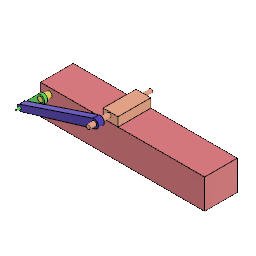
4 v1 (Autodesk Fusion 360 design; units mm, degrees)
Autodesk Fusion 360 part; units mm, degrees
sketch "Sketch1" plane through (0, 0, 0) normal (0, 1, 0) x (1, 0, 0)
  line L0 (0, -50) -> (150, -50)
  line L1 (150, -50) -> (150, 0)
  line L2 (150, 0) -> (0, 0)
  line L3 (0, 0) -> (0, -50)
  line L4 (125, -50) -> (150, -50)
  line L5 (150, -50) -> (150, -65)
  line L6 (150, -65) -> (125, -65)
  line L7 (125, -65) -> (125, -50)
  circle A0 centre (135, -60) radius 3.3426
  circle A1 centre (15, -40) radius 4.5426
  constraint horizontal L0
  constraint vertical L1
  constraint horizontal L2
  constraint vertical L3
  constraint horizontal L4
  constraint vertical L5
  constraint horizontal L6
  constraint vertical L7
  constraint coincident L0 L4.start
extrude "Extrude1" add sketch "Sketch1" along normal blind 55 contours L0 L1 L2 L3 L4 makes body 1 in component "Component"
extrude "Extrude1'" add sketch "Sketch1" along normal blind 55 separate body contours L0 L4 L5 L6 L7 makes body 2 in component "Component'"
extrude "Extrude1''" add sketch "Sketch1" along normal blind 60 and the other way blind 10 separate body contours A1 makes body 3 in component "Component''"
sketch "Sketch2" plane through (0, -10, 0) normal (0, -1, 0) x (1, 0, 0)
  circle A0 centre (15, 40) radius 4.5426
  circle A1 centre (15, 40) radius 7.2111
  circle A2 centre (15, 8.7998) radius 3.3899
  line L0 (7.8047, 40.4772) -> (11.634, 8.398)
  line L1 (22.1953, 40.4772) -> (18.366, 8.398)
  constraint concentric A0 A1
  constraint coincident A1 L0.start
  constraint coincident A2 L0.end
  constraint tangent A2 L0
  constraint coincident A1 L1.start
  constraint coincident A2 L1.end
  constraint tangent A2 L1
sketch "Sketch3" plane through (0, -10, 0) normal (0, -1, 0) x (1, 0, 0)
  circle A0 centre (15, 9) radius 1.6144
extrude "Extrude1'''" add sketch "Sketch2" along normal blind 5 separate body contours A1 L0 L1 | A1 A2 L0 L1 | A2 makes body 4 in component "Component'''"
extrude "Extrude2" cut sketch "Sketch3" along normal blind 10 bodies 4 in component "Component'''"
sketch "Sketch4" plane through (0, 0, 0) normal (0, 1, 0) x (1, 0, 0)
  circle A0 centre (135, -60) radius 80.8968
sketch "Sketch5" plane through (0, 0, 0) normal (0, 1, 0) x (1, 0, 0)
  circle A0 centre (135, -60) radius 7.074
  circle A1 centre (15, -9) radius 2.2361
  circle A2 centre (15, -9) radius 5.099
  circle A3 centre (135, -60) radius 4.1231
  line L0 (12.9347, -13.662) -> (132.1348, -66.4678)
  line L1 (137.668, -53.4484) -> (16.9231, -4.2775)
  constraint concentric A1 A2
  constraint concentric A0 A3
  constraint coincident A2 L0.start
  constraint coincident A0 L0.end
  constraint coincident A0 L1.start
  constraint coincident A2 L1.end
  constraint tangent A2 L1
  constraint tangent A0 L1
  constraint tangent A0 L0
  constraint tangent A2 L0
extrude "Extrude1''''" add sketch "Sketch5" along normal blind 10 separate body makes body 5
move_body "Move1" bodies 5 to x (1, 0, 0) y (0, 1, 0) z (0, 0, 1) at (0, -25, 0)
copy_body "Body->Comp1" bodies 5 removing the originals makes body 6 in component "Component''''"
extrude "Extrude2'" add sketch "Sketch1" along normal blind 70 and the other way blind 35 contours A0 bodies 2 in component "Component'"
extrude "Extrude3" add sketch "Sketch3" along normal blind 15 bodies 4 in component "Component'''"
extrude "Extrude4" add 1 faces at (15.4446, -25, 8.6969) along direction (0, -1, 0) blind 6.5 on bodies 4 bodies 4 in component "Component'''"
extrude "Extrude2''" add 1 faces at (150, 18.3333, 33.3333) along direction (1, 0, 0) blind 125 on bodies 1 bodies 1 in component "Component"
extrude "Extrude2'''" cut 1 faces at (16.4146, -10, 40.8776) along direction (0, 1, 0) blind 27 on bodies 3 bodies 3 in component "Component''"
component "Component" placed x (1, 0, 0) y (0, 1, 0) z (0, 0, 1) at (0, 0, 0)
component "Component'" placed x (1, 0, 0) y (0, 1, 0) z (0, 0, 1) at (6.8954, 0, 0)
component "Component''" placed x (-0.031862, 0, 0.999492) y (0, 1, 0) z (-0.999492, 0, -0.031862) at (55.4576, -32, 26.2821)
component "Component'''" placed x (0.977101, 0, 0.212778) y (0, 1, 0) z (-0.212778, 0, 0.977101) at (8.8546, 0, -2.2757)
component "Component''''" placed x (0.999983, 0, -0.005908) y (0, 1, 0) z (0.005908, 0, 0.999983) at (6.5432, 0, 0.7987)
